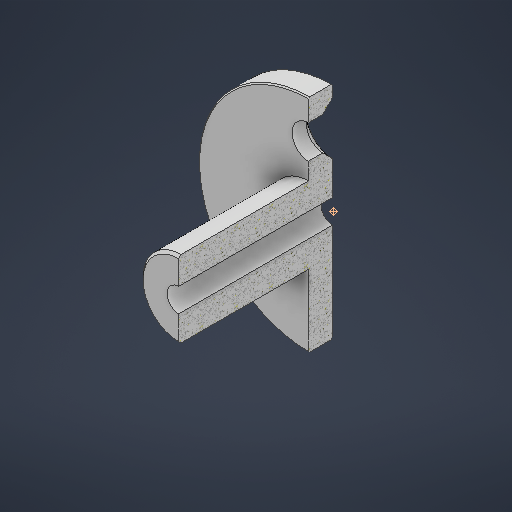
# Autodesk Inventor part: CylinderCover
Saved by Autodesk Inventor 2025.4 (Build 294407000, 407)
## iProperties
Created: 2026-05-29
Part Number: CylinderCover
Material: Generic
Document SubType Name: Modeling
Designer: VuQuan
Density: 1 g/cm^3
Appearance: Default
Author: VuQuan
Autodesk Inventor part; units mm, degrees
ref_plane "YZ Plane" through (0, 0, 0) normal (1, 0, 0) x (0, 1, 0)
ref_plane "XZ Plane" through (0, 0, 0) normal (0, 1, 0) x (-1, 0, 0)
ref_plane "XY Plane" through (0, 0, 0) normal (0, 0, 1) x (1, 0, 0)
sketch "Sketch1" plane through (0, 0, 0) normal (0, 0, 1) x (1, 0, 0)
  circle A0 centre (0, 0) radius 23
  circle A1 centre (0, 0) radius 8
  circle A2 centre (0, 0) radius 2.5
  circle A3 centre (0, 15) radius 3.5
  dimension "d0" = 46
  dimension "d1" = 16
  dimension "d2" = 5
  dimension "d3" = 7
  dimension "d4" = 15
  constraints: 4 centre point, 3 coincident, 1 vertical alignment
  measures "d0" diameter of A0
  measures "d1" diameter of A1
  measures "d2" diameter of A2
  measures "d3" diameter of A3
  measures "d4" distance of A3.centre point (0, 0)
extrude "Extrusion1" add sketch "Sketch1" along normal blind 5 contours A0
extrude "Extrusion2" add sketch "Sketch1" along normal blind 32 contours A1
chamfer "Chamfer1" distance 0.5 angle 45 1 edges at (-8, 0, 32)
chamfer "Chamfer2" distance 0.25 angle 45 2 edges at (-23, 0, 5) (-23, 0, 0)
chamfer "Chamfer3" distance 2 angle 45 1 edges at (-3.5, 15, 0)
body "Solid1"
